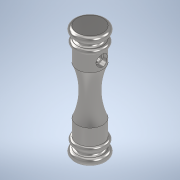
# Autodesk Inventor part: Wheel Shaft Pillar
Saved by Autodesk Inventor 2021.1 (Build 251245010, 245A)
## iProperties
Created: 2025-09-17
Part Number: Wheel Shaft Pillar
Material: Stainless Steel
Document SubType Name: Modeling
Designer: SD
Density: 8 g/cm^3
Appearance: Semi-Polished
Mass: 88.8009 g
Surface Area: 49.5731 cm^2
Volume: 11.1001 cm^3
Project: Automatic Tea Steeping mechanism
BOM-Mass: 0.08880
BOM-Area: 0.005
Length: 70.000 mm
Diameter: 20.000 mm
Author: SD
Title: Wheel Shaft Pillar
Autodesk Inventor part; units mm, degrees
ref_plane "XZ Plane" through (0, 0, 0) normal (0, 1, 0) x (-1, 0, 0)
sketch "Sketch1" plane through (0, 0, 0) normal (0, 0, 1) x (1, 0, 0)
  line L0 (0, 0) -> (0, -70)
  line L1 (0, 0) -> (8, 0)
  line L2 (8, 0) -> (8, -4) construction
  arc A0 (8, -4) -> (8, 0) centre (8, -2) ccw
  arc A1 (8, -4) -> (8, -7) centre (8, -5.5) ccw
  line L3 (8, -5.5) -> (4.7369, -5.5) construction
  arc A2 (8, -10) -> (8, -7) centre (8, -8.5) ccw
  line L4 (0, -70) -> (8, -70)
  line L5 (8, -70) -> (8, -66) construction
  arc A3 (8, -70) -> (8, -66) centre (8, -68) ccw
  arc A4 (8, -63) -> (8, -66) centre (8, -64.5) ccw
  arc A5 (8, -63) -> (8, -60) centre (8, -61.5) ccw
  arc A6 (8, -20) -> (8, -50) centre (45.081, -35) ccw
  line L6 (8, -10) -> (8, -20)
  line L7 (8, -50) -> (8, -60)
  dimension "d1" = 10
  dimension "d2" = 4
  dimension "d3" = 1.5
  dimension "d4" = 3
  dimension "d5" = 3
  dimension "d6" = 1.5
  dimension "d7" = 4
  dimension "d8" = 10
  dimension "d9" = 1.5
  dimension "d10" = 3
  dimension "d11" = 3
  dimension "d12" = 1.5
  dimension "d16" = 20
  dimension "d17" = 20
  dimension "d18" = 40
  dimension "d19" = 10
  dimension "d20" = 10
  constraints: 16 end point, 14 point on circle, 7 centre point, 5 vertical alignment, 3 horizontal, 3 vertical, 2 midpoint
  measures "d2" distance of L1.end L2.end
  measures "d3" radius of A1
  measures "d4" distance of A1.end L2.end
  measures "d5" distance of A1.end L6.start
  measures "d6" radius of A2
  measures "d7" distance of L4.end L5.end
  measures "d9" radius of A4
  measures "d10" distance of L5.end A4.start
  measures "d11" distance of A4.start L7.end
  measures "d12" radius of A5
  measures "d16" distance from line of L6.end L1
  measures "d17" distance from line of L7.start L4
  measures "d18" radius of A6
  measures "d19" distance of L6.start L6.end
  measures "d20" distance of L7.start L7.end
revolve "Revolution1" add sketch "Sketch1" angle 360 about axis through (0, 0, 0) along (0, -1, 0)
sketch "Sketch2" plane through (0, 0, 0) normal (1, 0, 0) x (0, 1, 0)
  circle A0 centre (-15, 0) radius 2.5
  line L0 (-70, 8) -> (-70, -8) projected
  point P0 (0, 0)
  dimension "d14" = 55
  dimension "d15" = 5
  constraints: 1 centre point, 1 horizontal alignment
  measures "d14" distance from line of L0 A0.centre
  measures "d15" diameter of A0
extrude "Extrusion1" cut sketch "Sketch2" against normal mid plane 20
ref_plane "Work Plane1" through (8, 0, 0) normal (1, 0, 0) x (0, 1, 0)
sketch "Sketch3" plane through (8, 0, 0) normal (1, 0, 0) x (0, 1, 0)
  spline S0 degree 7 poles (-12.5, 0) (-12.5, 0.2938) (-12.5403, 0.5803) (-12.6172, 0.8528) (-12.726, 1.106) (-12.8608, 1.3351) (-13.0141, 1.5373) (-13.3943, 1.9422) (-13.636, 2.1312) (-13.8942, 2.2799) (-14.1634, 2.3901) (-14.4396, 2.4633) (-14.7194, 2.5) (-15.2806, 2.5) (-15.5605, 2.4633) (-15.8366, 2.3901) (-16.1058, 2.2799) (-16.364, 2.1312) (-16.6057, 1.9422) (-16.9858, 1.5374) (-17.1392, 1.3352) (-17.274, 1.106) (-17.3828, 0.8528) (-17.4597, 0.5802) (-17.5, 0.2937) (-17.5, -0.2938) (-17.4597, -0.5803) (-17.3828, -0.8528) (-17.274, -1.106) (-17.1392, -1.3351) (-16.9859, -1.5373) (-16.6057, -1.9422) (-16.364, -2.1312) (-16.1058, -2.2799) (-15.8366, -2.3901) (-15.5605, -2.4633) (-15.2806, -2.5) (-14.7194, -2.5) (-14.4395, -2.4633) (-14.1634, -2.3901) (-13.8942, -2.2799) (-13.636, -2.1312) (-13.3943, -1.9422) (-13.0142, -1.5374) (-12.8608, -1.3352) (-12.726, -1.1059) (-12.6172, -0.8527) (-12.5403, -0.5801) (-12.5, -0.2937) (-12.5, 0) knots 0 0 0 0 0 0 0 0 0.107464 0.107464 0.107464 0.107464 0.107464 0.107464 0.249987 0.249987 0.249987 0.249987 0.249987 0.249987 0.392536 0.392536 0.392536 0.392536 0.392536 0.392536 0.499984 0.499984 0.499984 0.499984 0.499984 0.499984 0.607464 0.607464 0.607464 0.607464 0.607464 0.607464 0.750013 0.750013 0.750013 0.750013 0.750013 0.750013 0.892563 0.892563 0.892563 0.892563 0.892563 0.892563 1 1 1 1 1 1 1 1 projected
  circle A0 centre (-15, 0) radius 3.5
  line L0 (-70, 8) -> (-70, -8) projected
  point P0 (0, 0)
  dimension "d24" = 7
  dimension "d25" = 55
  constraints: 1 centre point, 1 horizontal alignment, 1 other
  measures "d24" diameter of A0
  measures "d25" distance from line of L0 A0.centre
extrude "Extrusion2" cut sketch "Sketch3" against normal blind 3
ref_plane "Work Plane2" through (-8, 0, 0) normal (1, 0, 0) x (0, 1, 0)
sketch "Sketch4" plane through (-8, 0, 0) normal (1, 0, 0) x (0, 1, 0)
  circle A0 centre (-15, 0) radius 2.5 projected
  circle A1 centre (-15, 0) radius 3.5
  point P0 (0, 0)
  dimension "d29" = 7
  constraints: 1 centre point, 1 coincident
  measures "d29" diameter of A1
extrude "Extrusion3" cut sketch "Sketch4" along normal blind 3
sketch "Sketch5" plane through (0, -70, 0) normal (0, -1, 0) x (1, 0, 0)
  point P0 (0, 0)
  point P1 (0, 0)
  constraints: 1 coincident
hole "Hole1" at (0, -70, 0) direction (0, 1, 0) diameter 6.647 depth 22.2 tip angle 118 thread size "M8x1.25" class "6H" standard "ISO Metric profile"
body "Solid1"
